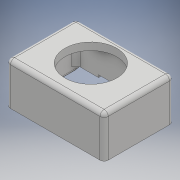
# Autodesk Inventor part: lupa-card-c-mount
Saved by Autodesk Inventor 2018 (Build 220112000, 112)
## iProperties
Created: 2018-03-09
Part Number: lupa-card-c-mount
Material: Generic
Document SubType Name: Modeling
Designer: matth
Density: 1 g/cm^3
Appearance: Default
Author: matth
Autodesk Inventor part; units mm, degrees
ref_plane "YZ Plane" through (0, 0, 0) normal (1, 0, 0) x (0, 1, 0)
ref_plane "XZ Plane" through (0, 0, 0) normal (0, 1, 0) x (-1, 0, 0)
ref_plane "XY Plane" through (0, 0, 0) normal (0, 0, 1) x (1, 0, 0)
sketch "Sketch1" plane through (0, 0, 0) normal (0, 0, 1) x (1, 0, 0)
  line L0 (-14.822, 23.7423) -> (29.878, 23.7423)
  line L1 (29.878, 23.7423) -> (29.878, -7.2577)
  line L2 (29.878, -7.2577) -> (-14.822, -7.2577)
  line L3 (-14.822, -7.2577) -> (-14.822, 23.7423)
  line L4 (31.278, 25.1423) -> (-16.222, 25.1423)
  line L5 (-16.222, 25.1423) -> (-16.222, -8.6577)
  line L6 (-16.222, -8.6577) -> (31.278, -8.6577)
  line L7 (31.278, -8.6577) -> (31.278, 25.1423)
  point P0 (0, 0)
  dimension "d0" = 44.7
  dimension "d1" = 31
  dimension "d2" = 1.4
  constraints: 16 end point, 4 parallel, 2 perpendicular, 1 horizontal, 3 other
  measures "d0" distance of L1.end L2.end
  measures "d1" distance of L2.end L0.start
  measures "d2" distance between parallel lines of L0 L4
extrude "Extrusion1" add sketch "Sketch1" along normal blind 17
sketch "Sketch2" plane through (0, 0, 17) normal (0, 0, 1) x (1, 0, 0)
  line L0 (31.278, 25.1423) -> (-16.222, 25.1423) projected
  line L1 (-16.222, 25.1423) -> (-16.222, -8.6577) projected
  line L2 (-16.222, -8.6577) -> (31.278, -8.6577) projected
  line L3 (31.278, -8.6577) -> (31.278, 25.1423) projected
  point P0 (0, 0)
extrude "Extrusion2" add sketch "Sketch2" along normal blind 1.4
sketch "Sketch4" plane through (0, 0, 17) normal (0, 0, -1) x (-1, 0, 0)
  circle A0 centre (-6.628, 9.5599) radius 12.6
  line L0 (-29.878, -7.2577) -> (-29.878, 23.7423) projected
  line L1 (14.822, 23.7423) -> (14.822, -7.2577) projected
  point P0 (0, 0)
  dimension "d7" = 23.25
  dimension "d8" = 44.7
  dimension "d9" = 25.2
  constraints: 1 centre point
  measures "d7" distance from line of L0 A0.centre
  measures "d8" distance between parallel lines of L0 L1
  measures "d9" diameter of A0
extrude "Extrusion3" cut sketch "Sketch4" against normal blind 1.4
sketch "Sketch5" plane through (0, 0, 17) normal (0, 0, -1) x (-1, 0, 0)
  circle A0 centre (-6.628, 9.5599) radius 12.6 projected
  circle A1 centre (-6.628, 9.5599) radius 14
  point P0 (0, 0)
  dimension "d12" = 1.4
  constraints: 1 centre point
  measures "d12" radial gap between concentric circles of A0 A1
extrude "Extrusion4" add sketch "Sketch5" along normal blind 2.2
chamfer "Chamfer1" distance 1 angle 45 1 edges at (20.628, 9.5599, 17)
sketch "Sketch6" plane through (0, 0, 0) normal (0, 0, -1) x (-1, 0, 0)
  line L0 (16.222, 25.1423) -> (16.222, -8.6577) projected
  line L1 (16.222, -8.6577) -> (-31.278, -8.6577) projected
  line L2 (-31.278, -8.6577) -> (-31.278, 25.1423) projected
  line L3 (14.822, 23.7423) -> (14.822, -7.2577) projected
  line L4 (14.822, -7.2577) -> (-29.878, -7.2577) projected
  line L5 (-29.878, -7.2577) -> (-29.878, 23.7423) projected
  line L6 (14.822, 23.7423) -> (-1.7434, 23.7423) projected
  line L7 (14.822, 23.7423) -> (14.822, 25.1423)
  line L8 (14.822, 25.1423) -> (16.222, 25.1423)
  line L9 (-29.878, 23.7423) -> (-29.878, 25.1423)
  line L10 (-29.878, 25.1423) -> (-31.278, 25.1423)
  point P0 (0, 0)
  constraints: 8 end point, 3 perpendicular, 1 point on line, 1 vertical
extrude "Extrusion5" add sketch "Sketch6" along normal blind 2
sketch "Sketch8" plane through (0, 0, -2) normal (0, 0, -1) x (-1, 0, 0)
  line L0 (14.822, -7.2577) -> (14.822, 23.7423) projected
  line L1 (-29.878, 23.7423) -> (-29.878, -7.2577) projected
  line L2 (14.822, -7.2577) -> (-29.878, -7.2577)
  line L3 (-29.878, -7.2577) -> (-29.878, 23.7423)
  line L4 (14.822, 23.7423) -> (14.822, -7.2577)
  line L5 (-29.678, -7.0577) -> (14.622, -7.0577)
  line L6 (14.622, -7.0577) -> (14.622, 23.5423)
  line L7 (-29.678, 23.5423) -> (-29.678, -7.0577)
  line L8 (14.622, 23.5423) -> (14.622, 23.7423)
  line L9 (-29.678, 23.5423) -> (-29.678, 23.7423)
  line L10 (-29.878, 23.7423) -> (14.822, 23.7423) projected
  line L11 (-29.878, 23.7423) -> (-29.678, 23.7423)
  line L12 (14.622, 23.7423) -> (14.822, 23.7423)
  point P0 (0, 0)
  dimension "d24" = 0.2
  constraints: 20 end point, 5 parallel, 4 perpendicular, 1 horizontal, 1 point on line, 1 other
  measures "d24" distance between parallel lines of L2 L5
extrude "Extrusion7" add sketch "Sketch8" against normal blind 0.4 contours L2 L1 L10 L9 L7 L5 L6 L8 L0
chamfer "Chamfer2" distance 0.2 angle 45 3 edges at (7.528, -7.0577, -1.6) (-14.622, 8.3423, -1.6) (29.678, 8.3423, -1.6)
chamfer "Chamfer3" distance 2 angle 45 1 edges at (-14.822, 23.7423, 8.5)
chamfer "Chamfer4" distance 2 angle 45 1 edges at (29.878, 23.7423, 8.5)
sketch "Sketch9" plane through (-14.822, 25.1423, 0) normal (0, 1, 0) x (1, 0, 0)
  line L0 (42.7, 0) -> (2, 0) projected
  line L1 (31.7, 0) -> (11, 0)
  line L2 (11, 0) -> (11, -1.2)
  line L3 (11, -1.2) -> (31.7, -1.2)
  line L4 (31.7, -1.2) -> (31.7, 0)
  line L5 (44.7, 0) -> (44.7, -17) projected
  line L6 (0, -17) -> (0, 0) projected
  point P0 (14.822, 0)
  dimension "d48" = 13
  dimension "d49" = 11
  dimension "d50" = 1.2
  constraints: 8 end point, 2 parallel, 1 horizontal, 1 perpendicular, 1 point on line
  measures "d48" distance between parallel lines of L5 L4
  measures "d49" distance between parallel lines of L6 L2
  measures "d50" distance between parallel lines of L0 L3
extrude "Extrusion8" cut sketch "Sketch9" against normal up to surface (1.4 mm away)
fillet "Fillet3" radius 2 8 edges at (7.528, 25.1423, 18.4) (-16.222, 8.2423, 18.4) (-16.222, 25.1423, 8.2) (-16.222, -8.6577, 8.2) (7.528, -8.6577, 18.4) (31.278, 8.2423, 18.4) (31.278, -8.6577, 8.2) (31.278, 25.1423, 8.2)
body "Solid1"
